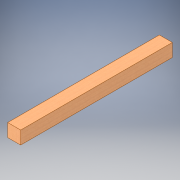
# Autodesk Inventor part: Столб-01
Saved by Autodesk Inventor 2019 (Build 230136000, 136)
## iProperties
Created: 2018-10-11
Part Number: Столб-01
Material: Дуб, красный
Document SubType Name: Modeling
Designer: Андреев Н.Л.
Density: 0.673 g/cm^3
Appearance: Вишневое дерево — натуральный — со слабым глянцем
ШИРИНА: 90
ТОЛЩВЫС: 90
ДЛИНА: 1050
Author: Андреев Н.Л.
Autodesk Inventor part; units mm, degrees
ref_plane "YZ Plane" through (0, 0, 0) normal (1, 0, 0) x (0, 1, 0)
ref_plane "XZ Plane" through (0, 0, 0) normal (0, 1, 0) x (-1, 0, 0)
ref_plane "XY Plane" through (0, 0, 0) normal (0, 0, 1) x (1, 0, 0)
sketch "Эскиз1" plane through (0, 0, 0) normal (0, 0, 1) x (1, 0, 0)
  line L0 (-45, -45) -> (45, -45)
  line L1 (45, -45) -> (45, 45)
  line L2 (45, 45) -> (-45, 45)
  line L3 (-45, 45) -> (-45, -45)
  line L4 (-45, -45) -> (45, 45) construction
  line L5 (45, -45) -> (-45, 45) construction
  point P0 (0, 0)
  dimension "ШИРИНА" = 90
  dimension "ТОЛЩВЫС" = 90
  constraints: 12 end point, 2 midpoint, 2 parallel, 1 horizontal, 1 perpendicular
  measures "ШИРИНА" distance of L2.end L1.end
  measures "ТОЛЩВЫС" distance of L1.end L0.end
extrude "Выдавливание1" add sketch "Эскиз1" along normal blind 1050
